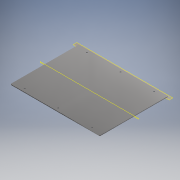
# Autodesk Inventor part: Deckel
Saved by Autodesk Inventor 2018 (Build 220112000, 112)
## iProperties
Created: 2017-10-08
Part Number: Deckel
Material: Edelstahl
Document SubType Name: Blech
Designer: jro
Density: 8 g/cm^3
Sheet Metal Rule: Standard_mm
Appearance: Halbpoliert
Author: jro
Autodesk Inventor part; units mm, degrees
ref_plane "YZ Plane" through (0, 0, 0) normal (1, 0, 0) x (0, 1, 0)
ref_plane "XZ Plane" through (0, 0, 0) normal (0, 1, 0) x (-1, 0, 0)
ref_plane "XY Plane" through (0, 0, 0) normal (0, 0, 1) x (1, 0, 0)
ref_plane "Arbeitsebene1" through (0, 0, 0) normal (0, 0, 1) x (1, 0, 0)
sketch "Skizze1" plane through (0, 0, 0) normal (0, 0, 1) x (1, 0, 0)
  line L0 (-141.4629, -2.7475) -> (141.4629, -2.7475)
  line L1 (141.4629, -6.7475) -> (-141.4629, -6.7475)
  arc A0 (-143.0858, -8.1175) -> (-141.4629, -6.7475) centre (-144.7619, -4.4856) ccw
  line L2 (-143.0858, -17.7475) -> (-143.0858, -8.1175)
  line L3 (143.0858, -17.7475) -> (-143.0858, -17.7475)
  line L4 (143.0858, -8.1175) -> (143.0858, -17.7475)
  arc A1 (141.4629, -6.7475) -> (143.0858, -8.1175) centre (144.7619, -4.4856) ccw
  line L5 (-141.4629, -218.7474) -> (141.4629, -218.7474)
  arc A2 (143.0858, -217.3774) -> (141.4629, -218.7474) centre (144.7619, -221.0093) ccw
  line L6 (143.0858, -207.7474) -> (143.0858, -217.3774)
  line L7 (-143.0858, -207.7474) -> (143.0858, -207.7474)
  line L8 (-143.0858, -217.3774) -> (-143.0858, -207.7474)
  arc A3 (-141.4629, -218.7474) -> (-143.0858, -217.3774) centre (-144.7619, -221.0093) ccw
  line L9 (146.5, -207.7104) -> (146.5, -217.7104)
  line L10 (146.5, -7.7845) -> (146.5, -17.7845)
  line L11 (-146.5, -216.7474) -> (-146.5, -8.7475)
  line L12 (146.5, -6.7475) -> (-146.5, -6.7475)
  line L13 (-146.5, -6.7475) -> (-146.5, -218.7474)
  line L14 (-146.5, -218.7474) -> (146.5, -218.7474)
  line L15 (146.5, -218.7474) -> (146.5, -6.7475)
  point P0 (0, 0)
  dimension "d0" = 0
  dimension "d1" = 0
  dimension "d2" = 0
  dimension "d3" = 0
  measures "d0" distance between parallel lines of L11 L13
  measures "d1" distance between parallel lines of L1 L12
  measures "d2" distance between parallel lines of L5 L14
  measures "d3" distance between parallel lines of L9 L15
extrude "Grobblech1" add sketch "Skizze1" along normal blind 2
ref_plane "Arbeitsebene3" through (-144.5, -112.7475, 0) normal (0, -1, 0) x (1, 0, 0)
sketch "Skizze2" plane through (0, 0, 2) normal (0, 0, 1) x (1, 0, 0)
  line L0 (-146.5, -6.7475) -> (146.5, -6.7475) projected
  line L1 (146.5, -218.7474) -> (-146.5, -218.7474) projected
  line L2 (141.4629, -224.7474) -> (-141.4629, -224.7474) projected
  line L3 (-141.4629, -0.7475) -> (141.4629, -0.7475) projected
  line L4 (146.5, -6.7475) -> (-146.5, -6.7475) projected
  line L5 (-146.5, -6.7475) -> (146.5, -6.7475)
  line L6 (146.5, -6.7475) -> (146.5, -0.7475)
  line L7 (146.5, -0.7475) -> (-146.5, -0.7475)
  line L8 (-146.5, -0.7475) -> (-146.5, -6.7475)
  line L9 (-146.5, -218.7474) -> (146.5, -218.7474)
  line L10 (146.5, -218.7474) -> (146.5, -224.7474)
  line L11 (146.5, -224.7474) -> (-146.5, -224.7474)
  line L12 (-146.5, -224.7474) -> (-146.5, -218.7474)
  point P0 (0, 0)
  constraints: 16 end point, 4 parallel, 2 horizontal, 2 perpendicular, 2 point on line
extrude "Extrusion1" add sketch "Skizze2" against normal up to surface (2 mm away)
fillet "Rundung1" radius 2 4 edges at (-146.5, -0.7475, 1) (146.5, -0.7475, 1) (146.5, -224.7474, 1) (-146.5, -224.7474, 1)
sketch "Skizze3" plane through (0, 0, 2) normal (0, 0, 1) x (1, 0, 0)
  circle A0 centre (-110, -10.7475) radius 1.65 construction
  circle A1 centre (0, -10.7475) radius 1.65 construction
  circle A2 centre (110, -10.7475) radius 1.65 construction
  circle A3 centre (-110, -214.7474) radius 1.65 construction
  circle A4 centre (0, -214.7474) radius 1.65 construction
  circle A5 centre (110, -214.7474) radius 1.65 construction
  circle A6 centre (110, -214.7474) radius 2.15
  circle A7 centre (0, -214.7474) radius 2.15
  circle A8 centre (-110, -214.7474) radius 2.15
  circle A9 centre (-110, -10.7475) radius 2.15
  circle A10 centre (0, -10.7475) radius 2.15
  circle A11 centre (110, -10.7475) radius 2.15
  point P0 (0, 0)
  dimension "d9" = 4.3
  dimension "d10" = 4.3
  dimension "d11" = 4.3
  dimension "d12" = 4.3
  dimension "d13" = 4.3
  dimension "d14" = 4.3
  constraints: 6 centre point, 6 coincident
  measures "d9" diameter of A6
  measures "d10" diameter of A7
  measures "d11" diameter of A8
  measures "d12" diameter of A9
  measures "d13" diameter of A10
  measures "d14" diameter of A11
extrude "Extrusion2" cut sketch "Skizze3" against normal through all
equation "\"d4\" = Stärke"
equation "\"Biegeradius\" = Stärke"
equation "\"BreiteBiegungsfreistellung\" = Stärke"
equation "\"TiefeBiegungsfreistellung\" = 0.5 * Stärke"
equation "\"GrößeEckenfreistellung\" = 4 * Stärke"
equation "\"MinimalRest\" = 2 * Stärke"
equation "\"Übergangsradius\" = Biegeradius"
equation "\"JacobiRadiusGröße\" = Biegeradius"
equation "\"Abstandsgröße\" = Stärke"
equation "\"Stärke\" = 2"
